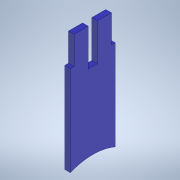
# Autodesk Inventor part: Paleta
Saved by Autodesk Inventor 2020.1 (Build 241239000, 239)
## iProperties
Created: 2020-03-26
Part Number: Paleta
Material: Laminate, Navy
Document SubType Name: Modeling
Designer: Daniel
Density: 1.38 g/cm^3
Appearance: Smooth - Navy
Author: Daniel
Autodesk Inventor part; units mm, degrees
ref_plane "YZ Plane" through (0, 0, 0) normal (1, 0, 0) x (0, 1, 0)
ref_plane "XZ Plane" through (0, 0, 0) normal (0, 1, 0) x (-1, 0, 0)
ref_plane "XY Plane" through (0, 0, 0) normal (0, 0, 1) x (1, 0, 0)
sketch "Sketch1" plane through (0, 0, 0) normal (1, 0, 0) x (0, 1, 0)
  circle A0 centre (-58.6732, 0) radius 31.02 construction
  line L0 (-39.6195, 0) -> (-14.1298, -32.6253) construction
  line L1 (-30.13, -12.146) -> (-30.13, 12.146) construction
  line L2 (0, 0) -> (-214.2426, 0) construction
  line L3 (-30.13, 12.146) -> (-33.107, -11.7755)
  line L4 (-33.107, -11.7755) -> (-30.13, -12.146)
  line L5 (-30.13, -12.146) -> (-27.153, 11.7755)
  line L6 (-27.153, 11.7755) -> (-30.13, 12.146)
  line L7 (-30.13, 12.146) -> (-30.13, -12.146) construction
  line L8 (-33.107, -11.7755) -> (-27.153, 11.7755) construction
  point P0 (-30.13, 0)
  dimension "d0" = 62.04
  dimension "d2" = 52
  dimension "d3" = 24.292
  dimension "d8" = 31.2206
  dimension "d9" = 16.0002
  dimension "d11" = 3
  dimension "d13" = 24.106
  constraints: 18 end point, 3 midpoint, 2 horizontal alignment, 2 parallel, 2 point on circle, 2 point on line, 1 centre point, 1 horizontal, 1 perpendicular, 1 vertical, 1 other
  measures "d0" diameter of A0
  measures "d2" angle of L2 L0
  measures "d3" distance of L1.start L1.end
  measures "d8" distance from line of L2.start L0
  measures "d9" distance from line of L0.end L1
  measures "d11" distance of L5.end L3.start
  measures "d13" distance of L3.start L3.end
sketch "Sketch2" plane through (0, 0, 0) normal (1, 0, 0) x (0, 1, 0)
  line L0 (0, 0) -> (63.4666, 0)
  line L1 (63.4666, 0) -> (63.4666, -24.106)
  line L2 (63.4666, -24.106) -> (0, -24.106)
  line L3 (0, -24.106) -> (0, 0) construction
  line L4 (63.4666, -12.053) -> (-45.5912, -12.053) construction
  arc A0 (0, -24.106) -> (0, 0) centre (-28.5826, -12.053) ccw
  arc A1 (0, 0) -> (0, -24.106) centre (-28.5826, -12.053) ccw construction
  line L5 (80.4558, -9.553) -> (46.4774, -9.553) construction
  line L6 (46.4774, -9.553) -> (46.4774, -14.553) construction
  line L7 (46.4774, -14.553) -> (80.4558, -14.553) construction
  line L8 (80.4558, -14.553) -> (80.4558, -9.553) construction
  line L9 (80.4558, -9.553) -> (46.4774, -14.553) construction
  line L10 (46.4774, -9.553) -> (80.4558, -14.553) construction
  line L11 (43.4774, -9.553) -> (83.4558, -9.553)
  line L12 (83.4558, -9.553) -> (83.4558, -14.553) construction
  line L13 (83.4558, -14.553) -> (43.4774, -14.553)
  line L14 (43.4774, -14.553) -> (43.4774, -9.553)
  line L15 (43.4774, -9.553) -> (83.4558, -14.553) construction
  line L16 (83.4558, -9.553) -> (43.4774, -14.553) construction
  line L17 (78.4666, -26.1591) -> (48.4666, -26.1591)
  line L18 (48.4666, -26.1591) -> (48.4666, -22.053)
  line L19 (48.4666, -22.053) -> (78.4666, -22.053)
  line L20 (78.4666, -22.053) -> (78.4666, -26.1591)
  line L21 (78.4666, -26.1591) -> (48.4666, -22.053) construction
  line L22 (48.4666, -26.1591) -> (78.4666, -22.053) construction
  line L23 (48.4666, 2.053) -> (48.4666, -2.053)
  line L24 (48.4666, -2.053) -> (78.4666, -2.053)
  point P0 (63.4666, -9.553)
  point P1 (63.4666, -2.053)
  point P2 (48.4666, 0)
  point P3 (48.4666, -24.106)
  point P4 (63.4666, -22.053)
  point P5 (63.4666, -14.553)
  dimension "d12" = 24.106
  dimension "d14" = 62.04
  dimension "d15" = 63.4666
  dimension "d17" = 109.0578
  dimension "d18" = 44.04
  dimension "d19" = 5
  dimension "d20" = 3
  dimension "d22" = 30
  dimension "d25" = 20
  constraints: 50 end point, 8 parallel, 7 midpoint, 5 horizontal, 4 perpendicular, 4 point on circle, 3 symmetric about line, 2 centre point, 1 collinear, 1 point on line
  measures "d12" distance of L2.end L0.start
  measures "d14" diameter of A0
  measures "d15" distance between parallel lines of L3 L1
  measures "d17" distance of L4.start L4.end
  measures "d18" distance edge to line of A0 L6
  measures "d19" distance of L7.end L5.start
  measures "d20" distance between parallel lines of L6 L14
  measures "d22" distance of L17.start L17.end
  measures "d25" distance between parallel lines of L24 L19
extrude "Extrusion1" add sketch "Sketch2" along normal blind 3 contours L0 L23 L24 L1 L11 L14 L13 L19 L18 L2 A0
equation "\"d12\" = d13"
body "Solid1"
